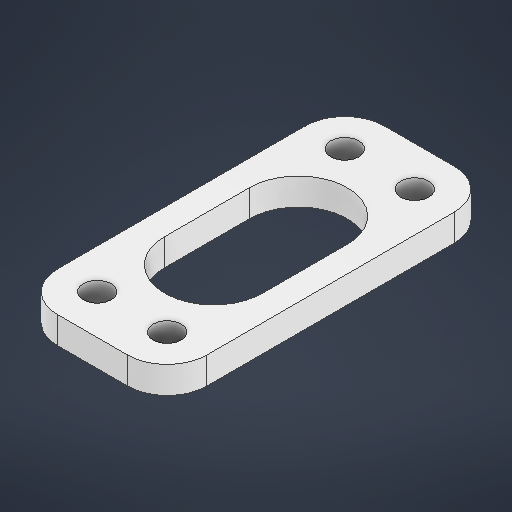
# Autodesk Inventor part: CNC-018-ZAxisBallScrewStabilizerShim1
Saved by Autodesk Inventor 2026.2 (Build 302298000, 298)
## iProperties
Created: 2026-06-22
Part Number: CNC-018-ZAxisBallScrewStabilizerShim1
Material: ABS Plastic
Document SubType Name: Modeling
Designer: Kenji
Density: 1.06 g/cm^3
Appearance: Smooth - White
Author: Kenji
Autodesk Inventor part; units mm, degrees
ref_plane "YZ Plane" through (0, 0, 0) normal (1, 0, 0) x (0, 1, 0)
ref_plane "XZ Plane" through (0, 0, 0) normal (0, 1, 0) x (-1, 0, 0)
ref_plane "XY Plane" through (0, 0, 0) normal (0, 0, 1) x (1, 0, 0)
sketch "Sketch1" plane through (0, 0, 0) normal (0, 1, 0) x (-1, 0, 0)
  circle A0 centre (0, 0) radius 2.6
  circle A1 centre (13, 0) radius 2.6
  circle A2 centre (13, 46) radius 2.6
  circle A3 centre (0, 46) radius 2.6
  circle A4 centre (13, 46) radius 7.3625 construction
  circle A5 centre (13, 0) radius 7.3625 construction
  circle A6 centre (0, 46) radius 7.3625 construction
  circle A7 centre (0, 0) radius 7.3625 construction
  line L0 (20.3625, 46) -> (20.3625, 0)
  line L1 (13, -7.3625) -> (0, -7.3625)
  line L2 (-7.3625, 0) -> (-7.3625, 46)
  line L3 (0, 53.3625) -> (13, 53.3625)
  arc A8 (13, -7.3625) -> (20.3625, 0) centre (13, 0) ccw
  arc A9 (-7.3625, 0) -> (0, -7.3625) centre (0, 0) ccw
  arc A10 (0, 53.3625) -> (-7.3625, 46) centre (0, 46) ccw
  arc A11 (20.3625, 46) -> (13, 53.3625) centre (13, 46) ccw
  line L4 (15.6, 45.6404) -> (15.6, 0) construction
  arc A12 (13, -2.6) -> (15.6, 0) centre (13, 0) ccw
  line L5 (13, -2.6) -> (0, -2.6) construction
  arc A13 (-2.6, 0) -> (0, -2.6) centre (0, 0) ccw
  line L6 (-2.6, 0) -> (-2.6, 46) construction
  arc A14 (0, 48.6) -> (-2.6, 46) centre (0, 46) ccw
  line L7 (0, 48.6) -> (13, 48.6) construction
  arc A15 (15.6, 46) -> (13, 48.6) centre (13, 46) ccw
  arc A16 (15.6, 30.8751) -> (-2.6, 30.8751) centre (6.5, 30.8751) ccw
  arc A17 (-2.6, 15.1249) -> (15.6, 15.1249) centre (6.5, 15.1249) ccw
  line L8 (15.6, 15.1249) -> (15.6, 30.8751)
  line L9 (-2.6, 30.8751) -> (-2.6, 15.1249)
  dimension "d0" = 5.2
  dimension "d1" = 13
  dimension "d2" = 46
  dimension "d3" = 4.7625
  dimension "d4" = 4.7625
  constraints: 29 point on circle, 20 end point, 18 centre point, 16 tangent, 8 equal radius, 4 coincident, 4 perpendicular, 4 point on line, 2 horizontal alignment, 2 vertical alignment, 1 collinear, 7 other
  measures "d0" diameter of A1
  measures "d1" distance of point (0, 0) A1.centre
  measures "d2" distance of A3.centre point (0, 0)
  measures "d3" radial gap between concentric circles of A4 A2
  measures "d4" distance between parallel lines of L4 L0
extrude "Extrusion1" add sketch "Sketch1" along normal blind 5
body "Solid1"
